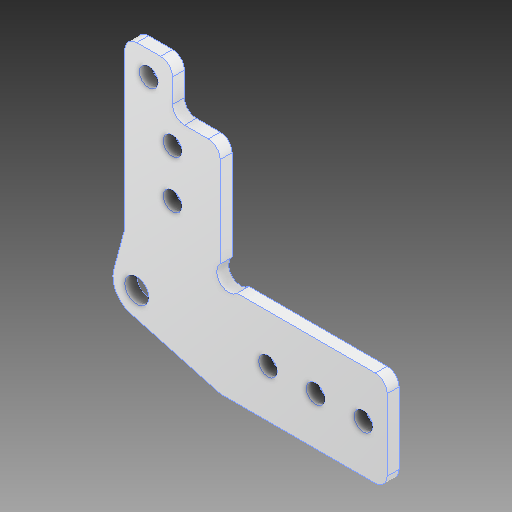
# Autodesk Inventor part: Bottom Bearing Plate (R4 - 0.25in Between Stages)
Saved by Autodesk Inventor 2022 (Build 260153000, 153)
## iProperties
Created: 2020-09-04
Part Number: Bottom Bearing Plate (R4 - 0.25in Between Stages)
Material: Aluminum 6061
Document SubType Name: Modeling
Density: 2.7 g/cm^3
Appearance: Aluminum - Flat
Autodesk Inventor part; units mm, degrees
ref_plane "YZ Plane" through (0, 0, 0) normal (1, 0, 0) x (0, 1, 0)
ref_plane "XZ Plane" through (0, 0, 0) normal (0, 1, 0) x (-1, 0, 0)
ref_plane "XY Plane" through (0, 0, 0) normal (0, 0, 1) x (1, 0, 0)
sketch "Sketch1" plane through (0, 0, 0) normal (0, 0, 1) x (1, 0, 0)
  line L0 (0, 0) -> (0, 13.4062)
  line L1 (0, 0) -> (20.3742, 0)
  circle A0 centre (9.525, 12.7) radius 9.525 construction
  circle A1 centre (9.525, 12.7) radius 3.2004
  line L2 (31.75, 0) -> (7.8407, 6.5775)
  arc A2 (3.3908, 14.3415) -> (7.8407, 6.5775) centre (9.525, 12.7) ccw
  line L3 (31.75, 0) -> (76.2, 0)
  line L4 (76.2, 0) -> (76.2, 25.4)
  line L5 (76.2, 25.4) -> (31.75, 25.4)
  line L6 (31.75, 25.4) -> (31.75, 57.15)
  line L7 (31.75, 57.15) -> (19.05, 57.15)
  line L8 (19.05, 57.15) -> (19.05, 69.85)
  line L9 (19.05, 69.85) -> (6.35, 69.85)
  line L10 (6.35, 69.85) -> (6.35, 25.4)
  line L11 (6.35, 25.4) -> (3.3908, 14.3415)
  circle A3 centre (12.7, 63.5) radius 2.4892
  line L12 (12.7, 69.85) -> (12.7, 63.5)
  circle A4 centre (44.45, 12.7) radius 2.4892
  circle A5 centre (57.15, 12.7) radius 2.4892
  circle A6 centre (69.85, 12.7) radius 2.4892
  circle A7 centre (19.05, 38.1) radius 2.4892
  circle A8 centre (19.05, 50.8) radius 2.4892
  line L13 (19.05, 50.8) -> (19.05, 38.1) construction
  arc A9 (31.75, 29.8901) -> (36.2401, 25.4) centre (33.9951, 27.6451) ccw
  circle A10 centre (31.2867, 27.5124) radius 0.4633 construction
  circle A11 centre (33.8624, 24.9367) radius 0.4633 construction
  line L14 (31.75, 25.4) -> (31.2867, 27.5124) construction
  line L15 (31.75, 25.4) -> (33.8624, 24.9367) construction
  point P0 (76.2, 12.7)
  dimension "d0" = 19.05
  dimension "d1" = 3.175
  dimension "d2" = 6.4008
  dimension "d6" = 12.7
  dimension "d7" = 25.4
  dimension "d8" = 4.9784
  dimension "d16" = 6.35
  dimension "d17" = 25.4
  dimension "d19" = 6.35
  dimension "d24" = 12.7
  dimension "d29" = 6.35
  dimension "d30" = 12.7
  dimension "d35" = 12.7
  dimension "d36" = 12.7
  dimension "d37" = 12.7
  dimension "d38" = 6.35
  dimension "d39" = 12.7
  dimension "d40" = 6.35
  constraints: 32 end point, 12 centre point, 7 tangent, 6 perpendicular, 5 point on circle, 4 equal radius, 4 vertical, 3 coincident, 3 horizontal, 3 vertical alignment, 2 horizontal alignment, 2 midpoint, 2 point on line, 1 collinear, 1 equal length, 5 other
  measures "d0" diameter of A0
  measures "d1" distance edge to line of A0 L1
  measures "d2" diameter of A1
  measures "d6" diameter of A2
  measures "d7" distance between parallel lines of L10 L6
  measures "d8" diameter of A3
  measures "d16" distance from line of L9 A3.centre
  measures "d17" distance between parallel lines of L3 L5
  measures "d19" distance between parallel lines of L0 L10
  measures "d24" distance of A4.centre A5.centre
  measures "d29" distance from line of A6.centre L4
  measures "d30" horizontal distance of L5.end A4.centre
  measures "d35" distance between parallel lines of L9 L7
  measures "d36" distance of L13.end L13.start
  measures "d37" distance from line of L5 L13.end
  measures "d38" distance from line of L7 L13.start
  measures "d39" distance between parallel lines of L10 L8
  measures "d40" diameter of A9
extrude "Extrusion1" add sketch "Sketch1" along normal blind 3.175 contours L2 A2 L11 L10 L9 L8 L7 L6 A9 L5 L4 L3
fillet "Fillet1" radius 3.175 8 edges at (6.35, 69.85, 1.5875) (19.05, 69.85, 1.5875) (76.2, 25.4, 1.5875) (76.2, 0, 1.5875) (6.35, 25.4, 1.5875) (31.75, 0, 1.5875) (31.75, 57.15, 1.5875) (19.05, 57.15, 1.5875)
equation "\"d24\" = d11"
equation "\"d11\" = 12.7"
body "Solid1"
